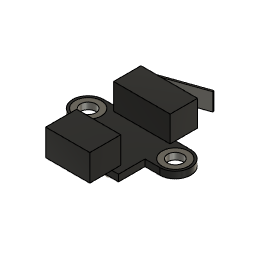
Z Endstop Mount v9 (Autodesk Fusion 360 archive; units mm, degrees)
design "Endstop"
Autodesk Fusion 360 part; units mm, degrees
sketch "PCB sketch" plane through (0, 0, 0) normal (0, 0, 1) x (1, 0, 0)
  line L0 (3.5, -3.5) -> (23.25, -3.5) construction
  arc A0 (23.25, -3.5) -> (23.25, 3.5) centre (23.25, 0) ccw
  line L1 (23.25, 3.5) -> (3.5, 3.5)
  arc A1 (3.5, 3.5) -> (3.5, -3.5) centre (3.5, 0) ccw
  line L2 (0, 0) -> (26.75, 0) construction
  line L3 (13.375, 3.5) -> (13.375, -9.5) construction
  line L4 (19.875, -9.5) -> (6.875, -9.5)
  line L5 (19.875, -9.5) -> (19.875, -3.5)
  line L6 (6.875, -9.5) -> (6.875, -3.5)
  line L7 (3.5, -3.5) -> (6.875, -3.5)
  line L8 (19.875, -3.5) -> (23.25, -3.5)
  circle A2 centre (23.25, 0) radius 1.75
  circle A3 centre (3.5, 0) radius 1.75
  circle A4 centre (3.5, 0) radius 3
  circle A5 centre (23.25, 0) radius 3
  dimension "d1" = 7
  dimension "d2" = 26.75
  dimension "d3" = 13
  dimension "d4" = 13
  dimension "d5" = 3.5
  dimension "d6" = 3.5
  dimension "d47" = 6
  dimension "d48" = 6
  constraint tangent L0 A0
  constraint tangent A0 L1
  constraint parallel L0 L1
  constraint tangent L1 A1
  constraint tangent L0 A1
  constraint midpoint A1 L2.start
  constraint midpoint A0 L2.end
  constraint horizontal L2
  constraint coincident L2.start origin
  constraint midpoint L1 L3.start
  constraint perpendicular L0 L3
  constraint perpendicular L3 L4
  constraint midpoint L3.end L4
  constraint coincident L0 L5.end
  constraint perpendicular L0 L5
  constraint coincident L0 L6.end
  constraint perpendicular L0 L6
  constraint concentric A0 A2
  constraint concentric A1 A3
  constraint concentric A1 A4
  constraint concentric A2 A5
  measures "d1" diameter of A0
  measures "d2" distance of L2.start L2.end
  measures "d3" distance of L3.start L3.end
  measures "d4" distance of L4.start L4.end
  measures "d5" diameter of A2
  measures "d6" diameter of A3
  measures "d47" diameter of A4
  measures "d48" diameter of A5
extrude "Extrude1" add sketch "PCB sketch" along normal blind 1.5 contours A0 L1 A1 L4 L5 L6 L7 L8 | A4 | A5 makes body 1
sketch "Connector Sketch" plane through (0, 0, 1.5) normal (0, 0, 1) x (-1, 0, 0)
  circle A0 centre (-23.25, 0) radius 1.75
  circle A1 centre (-3.5, 0) radius 1.75
  line L0 (-19.875, 9.5) -> (-19.875, 3.5)
  line L1 (-19.875, 3.5) -> (-23.25, 3.5)
  arc A2 (-23.25, 3.5) -> (-23.25, -3.5) centre (-23.25, 0) ccw
  line L2 (-23.25, -3.5) -> (-3.5, -3.5)
  arc A3 (-3.5, -3.5) -> (-3.5, 3.5) centre (-3.5, 0) ccw
  line L3 (-3.5, 3.5) -> (-6.875, 3.5)
  line L4 (-6.875, 3.5) -> (-6.875, 9.5)
  line L5 (-6.875, 9.5) -> (-19.875, 9.5) construction
  line L6 (-13.375, 9.5) -> (-13.375, -3.5) construction
  line L7 (-13.375, 9.5) -> (-13.375, 14.5) construction
  line L8 (-8.375, 14.5) -> (-18.375, 14.5)
  line L9 (-18.375, 14.5) -> (-18.375, 7.5)
  line L10 (-8.375, 14.5) -> (-8.375, 7.5)
  line L11 (-8.375, 7.5) -> (-18.375, 7.5)
  dimension "d9" = 5
  dimension "d10" = 10
  dimension "d11" = 7
  constraint midpoint L5 L6.start
  constraint midpoint L2 L6.end
  constraint perpendicular L5 L7
  constraint perpendicular L7 L8
  constraint midpoint L7.end L8
  constraint perpendicular L5 L9
  constraint perpendicular L5 L10
  constraint perpendicular L9 L11
  measures "d9" distance of L6.start L7.end
  measures "d10" distance of L8.start L8.end
  measures "d11" distance of L8.end L9.end
extrude "Extrude2" add sketch "Connector Sketch" along normal blind 6 contours L8 L9 L10 L11 bodies 1
sketch "Switch Sketch" plane through (0, 0, 1.5) normal (0, 0, 1) x (-1, 0, 0)
  line L0 (-18.375, 7.5) -> (-18.375, 9.5)
  line L1 (-18.375, 9.5) -> (-19.875, 9.5)
  line L2 (-19.875, 9.5) -> (-19.875, 3.5)
  line L3 (-19.875, 3.5) -> (-23.25, 3.5)
  arc A0 (-23.25, 3.5) -> (-23.25, -3.5) centre (-23.25, 0) ccw
  line L4 (-23.25, -3.5) -> (-3.5, -3.5) construction
  arc A1 (-3.5, -3.5) -> (-3.5, 3.5) centre (-3.5, 0) ccw
  line L5 (-3.5, 3.5) -> (-6.875, 3.5)
  line L6 (-6.875, 3.5) -> (-6.875, 9.5)
  line L7 (-6.875, 9.5) -> (-8.375, 9.5)
  line L8 (-8.375, 9.5) -> (-8.375, 7.5)
  line L9 (-8.375, 7.5) -> (-18.375, 7.5)
  circle A2 centre (-23.25, 0) radius 1.75
  circle A3 centre (-3.5, 0) radius 1.75
  line L10 (-19.775, -2.3) -> (-6.975, -2.3)
  line L11 (-6.975, -2.3) -> (-6.975, -8.5)
  line L12 (-6.975, -8.5) -> (-19.775, -8.5)
  line L13 (-19.775, -8.5) -> (-19.775, -2.3)
  line L14 (-13.375, -3.5) -> (-13.375, -8.5) construction
  dimension "d15" = 12.8
  dimension "d16" = 6.2
  dimension "d17" = 5
  constraint horizontal L10
  constraint vertical L11
  constraint horizontal L12
  constraint vertical L13
  constraint midpoint L4 L14.start
  constraint perpendicular L10 L14
  constraint midpoint L12 L14.end
  measures "d15" distance of L10.start L10.end
  measures "d16" distance of L10.start L12.end
  measures "d17" distance of L14.start L14.end
extrude "Extrude3" add sketch "Switch Sketch" along normal blind 5.85 contours L10 L11 L12 L13 bodies 1
sketch "Switch Button Sketch" plane through (0, 8.5, 0) normal (0, 1, 0) x (-1, 0, 0)
  line L0 (-19.775, 1.5) -> (-6.975, 1.5)
  line L1 (-6.975, 1.5) -> (-6.975, 7.35)
  line L2 (-6.975, 7.35) -> (-19.775, 7.35)
  line L3 (-19.775, 7.35) -> (-19.775, 1.5)
  line L4 (-6.975, 4.425) -> (-19.775, 4.425) construction
  line L5 (-10.825, 3) -> (-11.825, 3)
  line L6 (-11.825, 3) -> (-11.825, 5.85)
  line L7 (-11.825, 5.85) -> (-10.825, 5.85)
  line L8 (-10.825, 5.85) -> (-10.825, 3)
  line L9 (-10.825, 3) -> (-11.825, 5.85) construction
  line L10 (-11.825, 3) -> (-10.825, 5.85) construction
  point P0 (-11.325, 4.425)
  dimension "d20" = 1
  dimension "d21" = 2.85
  dimension "d22" = 3.85
  constraint midpoint L1 L4.start
  constraint midpoint L3 L4.end
  constraint horizontal L5
  constraint perpendicular L5 L6
  constraint parallel L5 L7
  constraint parallel L6 L8
  constraint coincident L9 P0
  constraint coincident L10 P0
  constraint coincident L4 P0
  measures "d20" distance of L6.end L7.end
  measures "d21" distance of L5.end L6.end
  measures "d22" distance of L1 L8
extrude "Extrude4" add sketch "Switch Button Sketch" along normal blind 1 contours L5 L6 L7 L8 bodies 1
ref_plane "WorkPlane1" through (13.375, 6, 4.425) normal (0, 0, -1) x (1, 0, 0)
sketch "Switch Arm Sketch" plane through (0, 0, 4.425) normal (0, 0, -1) x (-1, 0, 0)
  line L0 (-19.775, 8.5) -> (-6.975, 8.5)
  line L1 (-6.975, 8.5) -> (-7.975, 8.5)
  line L2 (-7.975, 8.5) -> (-7.8591, 8.8303) construction
  line L3 (-7.975, 8.5) -> (-19.2982, 12.4731)
  line L4 (-7.8591, 8.8303) -> (-19.1823, 12.8033)
  line L5 (-19.2982, 12.4731) -> (-19.1823, 12.8033)
  arc A0 (-7.625, 8.5) -> (-7.8591, 8.8303) centre (-7.975, 8.5) ccw
  point P0 (-6.975, 8.5)
  point P1 (-10.825, 9.5)
  dimension "d25" = 1
  dimension "d26" = 0.35
  dimension "d27" = 12
  dimension "d28" = 12
  dimension "d29" = 0.35
  constraint coincident P0 L0.end
  constraint parallel L0 L1
  constraint perpendicular L2 L3
  constraint perpendicular L2 L4
  constraint coincident L3 P1
  constraint coincident L0 A0.start
  constraint tangent L4 A0
  measures "d25" distance of P0 L1.end
  measures "d26" distance of L1.end L2.end
  measures "d27" distance of L1.end L3.end
  measures "d28" distance of L2.end L4.end
  measures "d29" radius of A0
extrude "Extrude5" add sketch "Switch Arm Sketch" along normal mid plane 4 separate body makes body 2
sketch "Soldered Pins Sketch" plane through (0, 0, 0) normal (0, 0, -1) x (1, 0, 0)
  circle A0 centre (23.25, 0) radius 1.75
  circle A1 centre (3.5, 0) radius 1.75
  line L0 (19.875, 3.5) -> (19.875, 9.5)
  line L1 (19.875, 9.5) -> (6.875, 9.5)
  line L2 (6.875, 9.5) -> (6.875, 3.5)
  line L3 (6.875, 3.5) -> (3.5, 3.5)
  arc A2 (3.5, 3.5) -> (3.5, -3.5) centre (3.5, 0) ccw
  line L4 (3.5, -3.5) -> (23.25, -3.5)
  arc A3 (23.25, -3.5) -> (23.25, 3.5) centre (23.25, 0) ccw
  line L5 (23.25, 3.5) -> (19.875, 3.5)
  line L6 (6.875, -1) -> (19.875, -1) construction
  line L7 (13.375, -3.5) -> (13.375, 9.5) construction
  line L8 (14.375, 0) -> (14.375, 1)
  arc A4 (14.375, 1) -> (12.375, 1) centre (13.375, 1) ccw
  line L9 (12.375, 1) -> (12.375, 0)
  arc A5 (12.375, 0) -> (14.375, 0) centre (13.375, 0) ccw
  line L10 (13.375, -1) -> (13.375, 2) construction
  line L11 (8.875, 0) -> (8.875, 1)
  arc A6 (8.875, 1) -> (6.875, 1) centre (7.875, 1) ccw
  line L12 (6.875, 1) -> (6.875, 0)
  arc A7 (6.875, 0) -> (8.875, 0) centre (7.875, 0) ccw
  line L13 (7.875, -1) -> (7.875, 2) construction
  line L14 (18.875, -1) -> (18.875, 2) construction
  arc A8 (19.875, 1) -> (17.875, 1) centre (18.875, 1) ccw
  line L15 (19.875, 1) -> (19.875, 0)
  arc A9 (17.875, 0) -> (19.875, 0) centre (18.875, 0) ccw
  line L16 (17.875, 0) -> (17.875, 1)
  line L17 (6.875, 9) -> (19.875, 9) construction
  line L18 (12.375, 8) -> (12.375, 7)
  arc A10 (12.375, 7) -> (14.375, 7) centre (13.375, 7) ccw
  line L19 (14.375, 7) -> (14.375, 8)
  arc A11 (14.375, 8) -> (12.375, 8) centre (13.375, 8) ccw
  line L20 (13.375, 9) -> (13.375, 6)
  line L21 (9.375, 8) -> (9.375, 7)
  arc A12 (9.375, 7) -> (11.375, 7) centre (10.375, 7) ccw
  line L22 (11.375, 7) -> (11.375, 8)
  arc A13 (11.375, 8) -> (9.375, 8) centre (10.375, 8) ccw
  line L23 (10.375, 9) -> (10.375, 6) construction
  arc A14 (17.375, 8) -> (15.375, 8) centre (16.375, 8) ccw
  line L24 (15.375, 7) -> (15.375, 8)
  line L25 (16.375, 9) -> (16.375, 6) construction
  arc A15 (15.375, 7) -> (17.375, 7) centre (16.375, 7) ccw
  line L26 (17.375, 8) -> (17.375, 7)
  point P0 (19.875, -1)
  dimension "d32" = 2.5
  dimension "d33" = 3
  dimension "d34" = 2
  dimension "d35" = 3
  dimension "d36" = 2
  dimension "d37" = 0.5
  dimension "d38" = 2
  dimension "d39" = 3
  dimension "d40" = 2
  dimension "d41" = 3
  dimension "d42" = 1
  constraint perpendicular L0 L6
  constraint midpoint L4 L7.start
  constraint perpendicular L4 L7
  constraint vertical L2.end L6.start
  constraint vertical L0.start P0
  constraint tangent L8 A4
  constraint tangent A4 L9
  constraint parallel L8 L9
  constraint tangent L9 A5
  constraint tangent L8 A5
  constraint midpoint A5 L10.start
  constraint midpoint A4 L10.end
  constraint perpendicular L6 L10
  constraint midpoint L6 L10.start
  constraint tangent L11 A6
  constraint tangent A6 L12
  constraint parallel L11 L12
  constraint tangent L12 A7
  constraint tangent L11 A7
  constraint midpoint A7 L13.start
  constraint midpoint A6 L13.end
  constraint perpendicular L6 L13
  constraint coincident L6 L13.start
  constraint collinear L2 L12
  constraint symmetric L6.start L7 P0
  constraint symmetric L7 L11.start A9.start
  constraint symmetric L7 L11.end A8.end
  constraint symmetric L7 A6.end A8.start
  constraint symmetric L7 L12.end L15.end
  constraint symmetric L7 A6 A8
  constraint symmetric L7 A7 A9
  constraint symmetric L7 L13.start L14.start
  constraint symmetric L7 L13.end L14.end
  constraint coincident L2 L17.start
  constraint coincident L0 L17.end
  constraint perpendicular L0 L17
  constraint tangent L18 A10
  constraint tangent A10 L19
  constraint parallel L18 L19
  constraint tangent L19 A11
  constraint tangent L18 A11
  constraint midpoint A11 L20.start
  constraint midpoint A10 L20.end
  constraint coincident L7 L20.end
  constraint perpendicular L17 L20
  constraint midpoint L17 L20.start
  constraint tangent L21 A12
  constraint tangent A12 L22
  constraint parallel L21 L22
  constraint tangent L22 A13
  constraint tangent L21 A13
  constraint midpoint A13 L23.start
  constraint midpoint A12 L23.end
  constraint perpendicular L17 L23
  constraint coincident L17 L23.start
  constraint symmetric L7 L21.start A14.start
  constraint symmetric L7 L21.end A15.end
  constraint symmetric L7 A12.end L24.start
  constraint symmetric L7 L22.end A14.end
  constraint symmetric L7 A12 A15
  constraint symmetric L7 A13 A14
  constraint symmetric L7 L23.start L25.start
  constraint symmetric L7 L23.end L25.end
  measures "d32" distance of L4 L6
  measures "d33" distance of L10.start L10.end
  measures "d34" diameter of A4
  measures "d35" distance of L13.start L13.end
  measures "d36" diameter of A6
  measures "d37" distance of L1 L17
  measures "d38" diameter of A10
  measures "d39" distance of L20.start L20.end
  measures "d40" diameter of A12
  measures "d41" distance of L23.start L23.end
  measures "d42" distance of L18 L22
extrude "Extrude6" add sketch "Soldered Pins Sketch" along normal blind 1.5 contours L8 A4 L9 A5 | L11 A6 L12 A7 | A8 L15 A9 L16 | L18 A10 A11 L20 | A10 L19 A11 L20 | L21 A12 L22 A13 | A14 L24 A15 L26 bodies 1
fillet "Fillet1" radius 1 24 edges at (16.375, -9, -1.5) (15.375, -7.5, -1.5) (16.375, -6, -1.5) (17.375, -7.5, -1.5) (13.375, -9, -1.5) (12.375, -7.5, -1.5) (13.375, -6, -1.5) (14.375, -7.5, -1.5) (10.375, -9, -1.5) (9.375, -7.5, -1.5) (10.375, -6, -1.5) (11.375, -7.5, -1.5) (8.875, -0.5, -1.5) (7.875, -2, -1.5) (6.875, -0.5, -1.5) (7.875, 1, -1.5) (14.375, -0.5, -1.5) (13.375, -2, -1.5) (12.375, -0.5, -1.5) (13.375, 1, -1.5) (18.875, -2, -1.5) (17.875, -0.5, -1.5) (18.875, 1, -1.5) (19.875, -0.5, -1.5) on bodies 1
combine "Combine1" operation add target body 1 tool bodies 2
split_face "SplitFace1" 2 faces at (15.5083, -1.5667, 1.5) (10.5818, -3.1112, 0) by curves path "PCB sketch" along A5 on bodies 1
split_face "SplitFace2" 2 faces at (11.3667, -0.4, 1.5) (10.5666, -3.121, 0) by curves path "PCB sketch" along A4 on bodies 1
copy_body "Body->Comp1" bodies 1 removing the originals makes body 3 in component "Endstop"
component "Endstop" placed x (1, 0, 0) y (0, 1, 0) z (0, 0, 1) at (0, 0, 0)
equation "d5 = 7 mm - ( ( 1.75 * 2 ) * 1 mm )"
named bodies: "Endstop", "Switch Arm"
